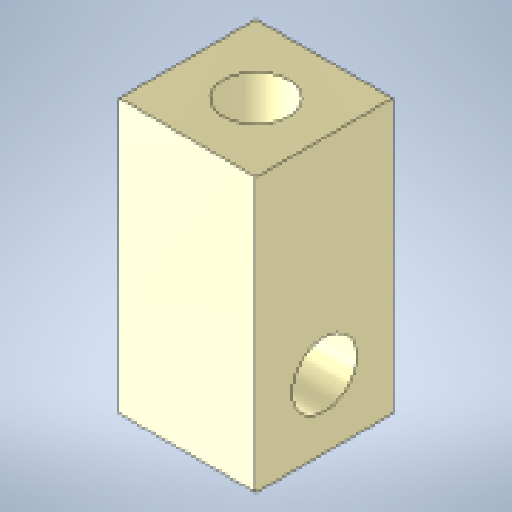
# Autodesk Inventor part: End Guides
Saved by Autodesk Inventor 2023.2 (Build 272271000, 271)
## iProperties
Created: 2024-02-24
Part Number: End Guides
Material: Nylon 6/6
Document SubType Name: Modeling
Designer: Nathan Cai
Density: 1.13 g/cm^3
Appearance: Nylon 6
Author: Nathan Cai
Autodesk Inventor part; units mm, degrees
ref_plane "YZ Plane" through (0, 0, 0) normal (1, 0, 0) x (0, 1, 0)
ref_plane "XZ Plane" through (0, 0, 0) normal (0, 1, 0) x (-1, 0, 0)
ref_plane "XY Plane" through (0, 0, 0) normal (0, 0, 1) x (1, 0, 0)
sketch "Sketch1" plane through (0, 0, 0) normal (1, 0, 0) x (0, 1, 0)
  line L0 (-4.7625, 3.175) -> (4.7625, 3.175)
  line L1 (4.7625, 3.175) -> (4.7625, -3.175)
  line L2 (4.7625, -3.175) -> (-4.7625, -3.175)
  line L3 (-4.7625, -3.175) -> (-4.7625, 3.175)
  line L4 (-4.7625, 3.175) -> (4.7625, -3.175) construction
  line L5 (4.7625, 3.175) -> (-4.7625, -3.175) construction
  line L6 (0, 3.175) -> (0, -3.175) construction
  line L7 (4.7625, 0) -> (-4.7625, 0) construction
  circle A0 centre (-1.5875, 0) radius 1.5
  point P0 (0, 0)
  dimension "d0" = 9.525
  dimension "d1" = 6.35
  dimension "d2" = 3
  dimension "d10" = 3.175
  constraints: 16 end point, 6 midpoint, 2 parallel, 1 centre point, 1 horizontal, 1 perpendicular, 1 point on line
  measures "d0" distance of L1.end L2.end
  measures "d1" distance of L0.end L1.end
  measures "d2" diameter of A0
  measures "d10" distance from line of L3 A0.centre
extrude "Extrusion1" add sketch "Sketch1" along normal blind 6.35
sketch "Sketch2" plane through (0, 4.7625, 3.175) normal (0, 1, 0) x (1, 0, 0)
  line L0 (0, 6.35) -> (0, 0) projected
  line L1 (0, 0) -> (6.35, 6.35) construction
  line L2 (6.35, 6.35) -> (6.35, 0) projected
  line L3 (6.35, 6.35) -> (6.35, 0)
  line L4 (0, 6.35) -> (6.35, 6.35) projected
  line L5 (6.35, 0) -> (0, 6.35) construction
  circle A0 centre (3.175, 3.175) radius 1.5
  point P0 (0, 3.175)
  dimension "d6" = 3
  constraints: 6 end point, 1 centre point, 1 collinear, 1 midpoint, 1 perpendicular
  measures "d6" diameter of A0
extrude "Extrusion2" cut sketch "Sketch2" against normal blind 6.35
fillet "Fillet1" radius 2.3813 1 edges at (6.35, -4.7625, 0)
fillet "Fillet2" radius 0.5 1 edges at (6.35, 4.7625, 0)
body "Solid1"
